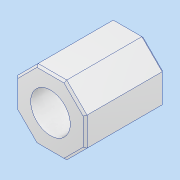
# Autodesk Inventor part: GearHub6kakku
Saved by Autodesk Inventor 2022 (Build 260153000, 153)
## iProperties
Created: 2024-04-30
Part Number: GearHub6kakku
Material: アルミニウム 6061
Document SubType Name: Modeling
Designer: ktamu
Density: 2.7 g/cm^3
Appearance: アルミニウム - フラット
Author: ktamu
Autodesk Inventor part; units mm, degrees
ref_plane "YZ Plane" through (0, 0, 0) normal (1, 0, 0) x (0, 1, 0)
ref_plane "XZ Plane" through (0, 0, 0) normal (0, 1, 0) x (-1, 0, 0)
ref_plane "XY Plane" through (0, 0, 0) normal (0, 0, 1) x (1, 0, 0)
sketch "スケッチ1" plane through (0, 0, 0) normal (0, 0, 1) x (1, 0, 0)
  circle A0 centre (0, 0) radius 2
  arc A1 (-3.5, 0) -> (-2.4749, -2.4749) centre (0, 0) ccw
  line L0 (-3.5, 3.5) -> (3.5, 3.5)
  line L1 (3.5, 3.5) -> (3.5, -3.5)
  line L2 (3.5, -3.5) -> (-3.5, -3.5)
  line L3 (-3.5, -3.5) -> (-3.5, 3.5)
  line L4 (-4.9497, 0) -> (0, 4.9497)
  line L5 (0, -4.9497) -> (-4.9497, 0)
  line L6 (4.9497, 0) -> (0, -4.9497)
  line L7 (0, 4.9497) -> (4.9497, 0)
  line L8 (-3.5, 1.4497) -> (-1.4497, 3.5)
  line L9 (1.4497, 3.5) -> (3.5, 1.4497)
  line L10 (3.5, -1.4497) -> (1.4497, -3.5)
  line L11 (-1.4497, -3.5) -> (-3.5, -1.4497)
  point P0 (-3.5, -1.4497)
  dimension "d0" = 4
  dimension "d1" = 7
  dimension "d2" = 7
  dimension "d3" = 7
  dimension "d6" = 45
  constraints: 24 end point, 15 point on line, 2 centre point, 2 coincident, 2 midpoint, 2 parallel, 2 perpendicular, 2 point on circle, 1 horizontal, 9 other
  measures "d0" diameter of A0
  measures "d1" diameter of A1
  measures "d2" distance of L1.end L2.end
  measures "d3" distance of L0.end L1.end
extrude "押し出し1" add sketch "スケッチ1" along normal blind 8 contours L3 L4 L0 L7 L1 L6 L2 L5 A1 | A1 L5 L3
chamfer "面取り1" distance 0.2 angle 45 8 edges at (-2.4749, 2.4749, 8) (0, 3.5, 8) (3.5, 0, 8) (0, -3.5, 8) (-2.4749, -2.4749, 8) (-3.5, 0, 8) (2.4749, 2.4749, 8) (2.4749, -2.4749, 8)
chamfer "面取り2" distance 0.2 angle 45 8 edges at (2.4749, 2.4749, 0) (3.5, 0, 0) (2.4749, -2.4749, 0) (0, 3.5, 0) (-2.4749, 2.4749, 0) (-3.5, 0, 0) (-2.4749, -2.4749, 0) (0, -3.5, 0)
